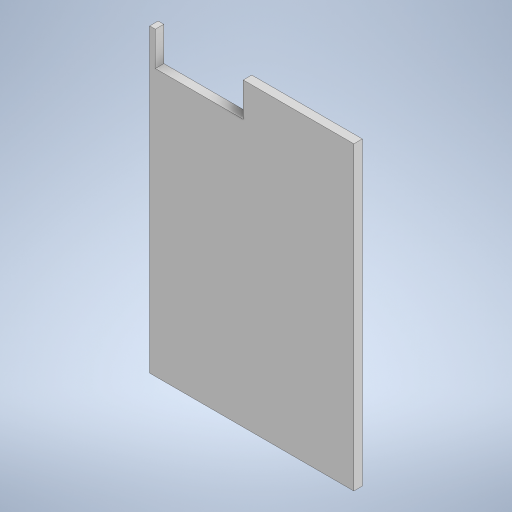
# Autodesk Inventor part: Lid
Saved by Autodesk Inventor 2024 (Build 280153000, 153)
## iProperties
Created: 2023-10-29
Part Number: Lid
Material: Generic
Document SubType Name: Modeling
Designer: zuhan
Density: 1 g/cm^3
Appearance: Default
Author: zuhan
Autodesk Inventor part; units mm, degrees
ref_plane "YZ Plane" through (0, 0, 0) normal (1, 0, 0) x (0, 1, 0)
ref_plane "XZ Plane" through (0, 0, 0) normal (0, 1, 0) x (-1, 0, 0)
ref_plane "XY Plane" through (0, 0, 0) normal (0, 0, 1) x (1, 0, 0)
sketch "Sketch1" plane through (0, 0, 0) normal (0, 0, 1) x (1, 0, 0)
  line L0 (-36, 53) -> (36, 53)
  line L1 (36, 53) -> (36, -53)
  line L2 (36, -53) -> (-36, -53)
  line L3 (-36, -53) -> (-36, 53)
  line L4 (-36, 53) -> (36, -53) construction
  line L5 (36, 53) -> (-36, -53) construction
  point P0 (0, 0)
  dimension "d0" = 72
  dimension "d1" = 106
  constraints: 12 end point, 2 midpoint, 2 parallel, 1 horizontal, 1 perpendicular
  measures "d0" distance of L1.end L2.end
  measures "d1" distance of L0.end L1.end
extrude "Extrusion1" add sketch "Sketch1" along normal blind 3
sketch "Sketch2" plane through (0, 0, 3) normal (0, 0, 1) x (1, 0, 0)
  line L0 (-34, 53) -> (4, 53)
  line L1 (4, 53) -> (4, 41)
  line L2 (4, 41) -> (-34, 41)
  line L3 (-34, 41) -> (-34, 53)
  line L4 (36, 53) -> (-36, 53) projected
  line L5 (-36, 53) -> (-36, -53) projected
  point P0 (0, 0)
  dimension "d4" = 0
  dimension "d5" = 2
  dimension "d6" = 12
  dimension "d7" = 38
  constraints: 8 end point, 2 parallel, 1 horizontal, 1 perpendicular
  measures "d4" distance between parallel lines of L4 L0
  measures "d5" distance between parallel lines of L5 L3
  measures "d6" distance between parallel lines of L0 L2
  measures "d7" distance between parallel lines of L3 L1
extrude "Extrusion2" cut sketch "Sketch2" against normal blind 3
sketch "Sketch3" plane through (4, 41, 3) normal (-1, 0, 0) x (0, 0, 1)
  point P0 (-3, -41)
sketch "Sketch7" plane through (-34, 41, 3) normal (0, 1, 0) x (1, 0, 0)
  line L0 (38, 3) -> (38, 0) projected
  line L1 (38, 3) -> (31, 3)
  line L2 (31, 3) -> (31, 0)
  line L3 (31, 0) -> (38, 0)
  line L4 (38, 0) -> (38, 3)
  point P0 (34, 3)
  dimension "d18" = 7
  dimension "d19" = 3
  constraints: 8 end point, 2 parallel, 1 horizontal, 1 perpendicular
  measures "d18" distance of L3.end L2.end
  measures "d19" distance of L2.end L1.end
extrude "Extrusion5" add sketch "Sketch7" along normal blind 12
body "Solid1"
